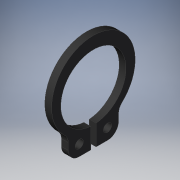
# Autodesk Inventor part: STWS10
Saved by Autodesk Inventor 2019 (Build 230136000, 136)
## iProperties
Created: 2022-11-16
Part Number: STWS10
Material: Generic
Catalog Web Link: www.cadenas.de
Description: STWN, STWS-Retaining Rings - C - External
Vendor: MISUMI
Document SubType Name: Modeling
Designer: psAdmin
Manufacturer: MISUMI
Mass: 0.0592753 g
Surface Area: 2.03896 cm^2
Volume: 0.0592753 cm^3
Density: 1 g/cm^3
Appearance: PSOLRGB-175-175-175
Category: PARTsolutions
Company: MISUMI
Title: STWS10
Author: Cadenas PARTsolutions
Comments: Retaining Rings - C - External
PSOL_IDENT_0: {$CADENAS_DATA/23d-libs/misumi/metric/28_keys_magnets/stwn.prj},159 {VTYP=3D},{NB=STWS10},{LINA=STWS
PSOL_IDENT_1: 10},{NN=STWN, STWS},{DATE=30.06.2021 13:10:01},{GEOMDATE=19.07.2012 00:00:00},{VERSION=},{LINEID=70}
PSOL_IDENT_2: ,{WBVAR=MAT},{WBNUMERIC=}  {NB=STWS10},{LINA=STWS10},{KT=DUMMY},{PN=STWS10},{TYPE=STWS},{MAT=2},{HAR
PSOL_IDENT_3: D=36~44HRC},{NO=10},{MATALG='1','Spring Steel','2','304 Stainless Steel-CSP'},{DD3=9.3},{DD3TOL=+0.1
PSOL_IDENT_4: 5/-0.15},{TT=1.00},{TTTOL=+0.05/-0.05},{BB=1.8},{AA=3.0},{DD0=1.2},{DD4=17.0},{DD1=10},{DD2=9.60},{D
PSOL_IDENT_5: D2TOL=0/-0.09},{MM=1.15},{MMTOL=+0.14/0},{NN=1.5},{H1=1.6},{A3=0.80},{A2=4.15},{A1=7.40},{R2=1.60},{
PSOL_IDENT_6: R1=1.60}
NB: STWS10
NN: 1.5
NT: Retaining Rings - C - External
NBSYN: $PN.
LINA: STWS10
CATALOG: Misumi
PN: STWS10
MAT: 304 Stainless Steel-CSP
HARD: 36~44HRC
NO: 10
DD3: 9.3
DD3TOL: +0.15/-0.15
TT: 1
TTTOL: +0.05/-0.05
BB: 1.8
AA: 3
DD0: 1.2
DD4: 17
DD1: 10
DD2: 9.6
DD2TOL: 0/-0.09
MM: 1.15
MMTOL: +0.14/0
SUPPLIER: MISUMI
ARTICLENO: STWS10
BOMINFO: STWS10
CREATOR: CADENAS GmbH
Autodesk Inventor part; units mm, degrees
sketch "Sketch_5" plane through (0, 0, 0) normal (1, 0, 0) x (0, 1, 0)
  arc A0 (-4.0371, -4.2058) -> (-4.0371, 4.2058) centre (0.45, 0) ccw
  arc A1 (-5.2044, 3.7) -> (-4.0371, 4.2058) centre (-5.2044, 5.3) ccw
  line L0 (-5.2044, 3.7) -> (-6.2, 3.7)
  arc A2 (-6.2, 3.7) -> (-7.8, 2.1) centre (-6.2, 2.1) ccw
  line L1 (-7.8, 2.1) -> (-7.8, 0.4)
  line L2 (-7.8, 0.4) -> (-6.8, 0.4)
  line L3 (-6.8, 0.4) -> (-6.8, 2.075)
  arc A3 (-5.6, 2.075) -> (-6.8, 2.075) centre (-6.2, 2.075) ccw
  line L4 (-5.6, 2.075) -> (-5.6, 0.4)
  line L5 (-5.6, 0.4) -> (-4.7833, 0.4)
  arc A4 (-4.7833, -0.4) -> (-4.7833, 0.4) centre (0, 0) ccw
  line L6 (-4.7833, -0.4) -> (-5.6, -0.4)
  line L7 (-5.6, -0.4) -> (-5.6, -2.075)
  arc A5 (-6.8, -2.075) -> (-5.6, -2.075) centre (-6.2, -2.075) ccw
  line L8 (-6.8, -2.075) -> (-6.8, -0.4)
  line L9 (-6.8, -0.4) -> (-7.8, -0.4)
  line L10 (-7.8, -0.4) -> (-7.8, -2.1)
  arc A6 (-7.8, -2.1) -> (-6.2, -3.7) centre (-6.2, -2.1) ccw
  line L11 (-6.2, -3.7) -> (-5.2044, -3.7)
  arc A7 (-4.0371, -4.2058) -> (-5.2044, -3.7) centre (-5.2044, -5.3) ccw
  constraints: 24 end point, 16 point on circle, 8 centre point
extrude "Extrusion1" add sketch "Sketch_5" along normal mid plane 1
sketch "Sketch_6" plane through (0, 0, 0) normal (1, 0, 0) x (0, 1, 0)
  arc A0 (-4.0371, -4.2058) -> (-4.0371, 4.2058) centre (0.45, 0) ccw
  arc A1 (-5.2044, 3.7) -> (-4.0371, 4.2058) centre (-5.2044, 5.3) ccw
  line L0 (-5.2044, 3.7) -> (-6.2, 3.7)
  arc A2 (-6.2, 3.7) -> (-7.8, 2.1) centre (-6.2, 2.1) ccw
  line L1 (-7.8, 2.1) -> (-7.8, 0.4)
  line L2 (-7.8, 0.4) -> (-4.7833, 0.4)
  arc A3 (-4.7833, -0.4) -> (-4.7833, 0.4) centre (0, 0) ccw
  line L3 (-4.7833, -0.4) -> (-7.8, -0.4)
  line L4 (-7.8, -0.4) -> (-7.8, -2.1)
  arc A4 (-7.8, -2.1) -> (-6.2, -3.7) centre (-6.2, -2.1) ccw
  line L5 (-6.2, -3.7) -> (-5.2044, -3.7)
  arc A5 (-4.0371, -4.2058) -> (-5.2044, -3.7) centre (-5.2044, -5.3) ccw
  circle A6 centre (-6.2, -2.075) radius 0.6
  circle A7 centre (-6.2, 2.075) radius 0.6
  constraints: 12 end point, 12 point on circle, 8 centre point
extrude "Extrusion2" add sketch "Sketch_6" along normal mid plane 1
ref_plane "1_XY" through (0, 0, 0) normal (1, 0, 0) x (0, 0, -1)
ref_plane "1_YZ" through (0, 0, 0) normal (0, 0, -1) x (0, 1, 0)
ref_plane "1_ZX" through (0, 0, 0) normal (0, 1, 0) x (1, 0, 0)
ref_plane "combination_module_XY" through (0.5, 0, 0) normal (1, 0, 0) x (0, 0, -1)
ref_plane "combination_module_YZ" through (0.5, 0, 0) normal (0, 0, -1) x (0, 1, 0)
ref_plane "combination_module_ZX" through (0.5, 0, 0) normal (0, 1, 0) x (1, 0, 0)
body "Solid1"
